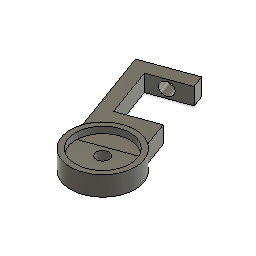
PL_StationaryPedestal (Autodesk Fusion 360 design; units mm, degrees)
Autodesk Fusion 360 part; units mm, degrees
sketch "Sketch1" plane through (0, 0, 0) normal (0, 1, 0) x (1, 0, 0)
  circle A0 centre (0, 0) radius 25
  dimension "d1" = 50
  constraint coincident A0.centre origin
  measures "d1" diameter of A0
extrude "Extrude1" add sketch "Sketch1" along normal blind 10
sketch "Sketch2" plane through (0, 10, 0) normal (0, 1, 0) x (-1, 0, 0)
  circle A0 centre (0, 0) radius 25
  circle A1 centre (0, 0) radius 21
  dimension "d4" = 42
  constraint coincident A0.centre A1.centre
  measures "d4" diameter of A1
extrude "Extrude2" cut sketch "Sketch2" against normal blind 5 contours A1
sketch "Sketch3" plane through (0, 5, 0) normal (0, 1, 0) x (-1, 0, 0)
  circle A0 centre (0, 0) radius 21
  circle A1 centre (0, 0) radius 5
  dimension "d7" = 10
  constraint coincident A0.centre A1.centre
  measures "d7" diameter of A1
extrude "Extrude3" cut sketch "Sketch3" against normal through all contours A1
ref_plane "WorkPlane1" through (-8.5505, 3.5882, -23.4923) normal (-0.34202, 0, -0.939693) x (0.939693, 0, -0.34202)
sketch "Sketch4" plane through (-8.5505, 3.5882, -23.4923) normal (-0.34202, 0, -0.939693) x (0.939693, 0, -0.34202)
  line L0 (-19.8743, 2.2343) -> (20.1257, 2.2343)
  line L1 (20.1257, 2.2343) -> (20.1257, -5.7657)
  line L2 (20.1257, -5.7657) -> (-19.8743, -5.7657)
  line L3 (-19.8743, -5.7657) -> (-19.8743, 2.2343)
  line L4 (-19.8743, 2.2343) -> (20.1257, -5.7657) construction
  line L5 (20.1257, 2.2343) -> (-19.8743, -5.7657) construction
  point P0 (0.1257, -1.7657)
  dimension "d10" = 40
  dimension "d11" = 8
  constraint horizontal L0
  constraint perpendicular L0 L1
  constraint parallel L0 L2
  constraint parallel L1 L3
  constraint coincident L4 P0
  constraint coincident L5 P0
  measures "d10" distance of L1.end L2.end
  measures "d11" distance of L0.end L1.end
extrude "Extrude4" add sketch "Sketch4" along normal blind 50 and the other way blind 17
extrude "Extrude5" cut 1 faces at (-6.1758, 9.3539, -10.4946) along direction (0, -1, 0) blind 4
extrude "Extrude6" add 1 faces at (-6.1758, 5.3539, -10.4946) along direction (0, -1, 0) blind 5
extrude "Extrude7" cut 1 faces at (-6.1758, 5.3539, -10.4946) along direction (0, -1, 0) blind 0.354
extrude "Extrude8" add 1 faces at (-19.2688, 6.6872, -72.8001) along direction (-0.34202, 0, -0.939693) blind 10
sketch "Sketch5" plane through (0, 9.3539, 0) normal (0, 1, 0) x (-1, 0, 0)
  arc A0 (-13.8395, -20.8199) -> (23.8629, -7.4541) centre (0, 0) ccw
  line L0 (-13.8395, -20.8199) -> (10.1597, -86.757)
  line L1 (10.1597, -86.757) -> (47.7474, -73.0762)
  line L2 (47.7474, -73.0762) -> (23.8629, -7.4541)
  line L3 (10.1597, -86.757) -> (6.7395, -77.36)
  line L4 (34.9302, -67.0994) -> (28.0898, -48.3056)
  line L5 (28.0898, -48.3056) -> (-0.1009, -58.5662)
  line L6 (34.9302, -67.0994) -> (6.7395, -77.36)
  dimension "d24" = 10
  dimension "d26" = 20
  constraint coincident L0.end L1.start
  constraint perpendicular L1 L3
  constraint coincident L0 L5.end
  constraint perpendicular L0 L5
  constraint perpendicular L0 L6
  measures "d24" distance of L0.end L3.end
  measures "d26" distance of L4.start L4.end
extrude "Extrude9" cut sketch "Sketch5" against normal through all contours L0 L4 L5 L6
extrude "Extrude10" add 1 faces at (-11.2915, 9.3539, -43.723) along direction (0, 1, 0) blind 5
extrude "Extrude11" add 1 faces at (-16.1839, 10, -17.1464) along direction (0, 1, 0) blind 5
extrude "Extrude12" add 1 faces at (-8.8107, 5, 12.8559) along direction (0, 1, 0) blind 5
extrude "Extrude13" add 1 faces at (-6.1758, 4.9999, -10.4946) along direction (0, 1, 0) blind 5
extrude "Extrude14" cut 1 faces at (-18.6929, 10.0206, -51.7258) along direction (0.34202, 0, 0.939693) blind 20
hole "Hole1" at (-25.5993, 7.935, -81.1374) direction (0.34202, 0, 0.939693) diameter 10 depth 14 tip angle 118
